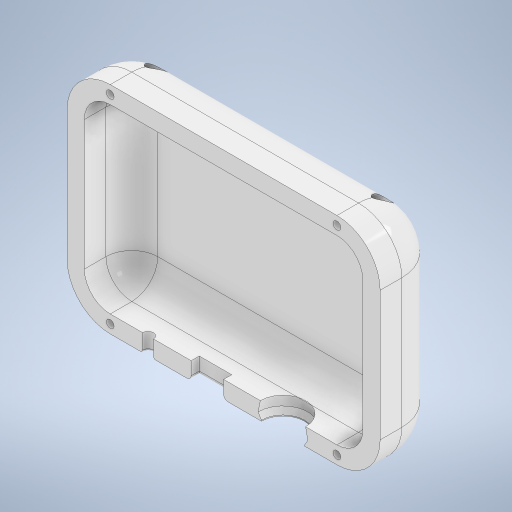
# Autodesk Inventor part: Case inferiore
Saved by Autodesk Inventor 2023 (Build 270158000, 158)
## iProperties
Created: 2022-12-30
Part Number: Case inferiore
Material: Plastica ABS
Document SubType Name: Modeling
Designer: Gabriele
Density: 1.06 g/cm^3
Appearance: Bianco
Author: Gabriele
Autodesk Inventor part; units mm, degrees
ref_plane "YZ Plane" through (0, 0, 0) normal (1, 0, 0) x (0, 1, 0)
ref_plane "XZ Plane" through (0, 0, 0) normal (0, 1, 0) x (-1, 0, 0)
ref_plane "XY Plane" through (0, 0, 0) normal (0, 0, 1) x (1, 0, 0)
sketch "Schizzo1" plane through (0, 0, 0) normal (0, 0, 1) x (1, 0, 0)
  line L0 (-52.5, -50) -> (52.5, -50)
  line L1 (72.5, -30) -> (72.5, 30)
  line L2 (52.5, 50) -> (-52.5, 50)
  line L3 (-72.5, 30) -> (-72.5, -30)
  line L4 (-72.5, -50) -> (72.5, 50) construction
  line L5 (72.5, -50) -> (-72.5, 50) construction
  arc A0 (-52.5, 50) -> (-72.5, 30) centre (-52.5, 30) ccw
  arc A1 (-72.5, -30) -> (-52.5, -50) centre (-52.5, -30) ccw
  arc A2 (52.5, -50) -> (72.5, -30) centre (52.5, -30) ccw
  arc A3 (72.5, 30) -> (52.5, 50) centre (52.5, 30) ccw
  point P0 (0, 0)
  dimension "d0" = 145
  dimension "d1" = 100
  dimension "d2" = 20
  constraints: 12 end point, 8 point on circle, 8 point on line, 8 tangent, 4 centre point, 3 equal radius, 2 midpoint, 2 parallel, 1 horizontal, 1 perpendicular
  measures "d0" distance of L4.end L5.end
  measures "d1" distance of L5.end L4.start
  measures "d2" radius of A0
extrude "Estrusione1" add sketch "Schizzo1" along normal blind 30
fillet "Raccordo1" radius 20 8 edges at (-66.6421, 44.1421, 0) (-72.5, 0, 0) (-66.6421, -44.1421, 0) (0, -50, 0) (66.6421, -44.1421, 0) (72.5, 0, 0) (66.6421, 44.1421, 0) (0, 50, 0)
shell "Svuotamento1" thickness 8 removed faces 1 at (17.5, 16.6667, 30)
sketch "Schizzo5" plane through (-52.5, -50, 30) normal (0, -1, 0) x (1, 0, 0)
  line L0 (52.5, 3.75) -> (37.5, 3.75)
  line L1 (37.5, 3.75) -> (37.5, -3.75)
  line L2 (37.5, -3.75) -> (52.5, -3.75)
  line L3 (52.5, -3.75) -> (52.5, 3.75)
  line L4 (105, 0) -> (0, 0) projected
  line L5 (52.5, 3.75) -> (37.5, -3.75) construction
  line L6 (37.5, 3.75) -> (52.5, -3.75) construction
  circle A0 centre (80, 0) radius 10
  circle A1 centre (17.5, 0) radius 2.55
  line L7 (0, 0) -> (105, 0) projected
  point P0 (52.5, -30)
  point P1 (52.5, 0)
  point P2 (52.5, 0)
  point P3 (70, 0)
  point P4 (90, 0)
  point P5 (52.5, 0)
  point P6 (37.5, 0)
  point P7 (14.95, 0)
  point P8 (20.05, 0)
  point P9 (45, 0)
  dimension "d16" = 5.1
  dimension "d17" = 15
  dimension "d19" = 20
  dimension "d28" = 3.75
  dimension "d29" = 7.5
  dimension "d78" = 25
  dimension "d79" = 27.5
  dimension "d80" = 17.5
  constraints: 12 end point, 4 point on line, 3 midpoint, 2 centre point, 2 parallel, 1 horizontal, 1 perpendicular
  measures "d16" diameter of A1
  measures "d17" distance of L0.start L0.end
  measures "d19" diameter of A0
  measures "d28" distance between parallel lines of L4 L2
  measures "d29" distance between parallel lines of L2 L0
  measures "d78" distance of L4.start A0.centre
  measures "d79" horizontal distance of L0.start A0.centre
  measures "d80" distance of L4.end A1.centre
extrude "Estrusione3" cut sketch "Schizzo5" against normal blind 9 contours L3 L2 L1 L4 | A0 L4 | A1 L4 picked at (77.0485, -1.5491) picked at (16.9445, -1.298)
sketch "Schizzo10" plane through (0, 0, 0) normal (0, 0, -1) x (-1, 0, 0)
  line L0 (52.5, 50) -> (-52.5, 50) projected
  line L1 (-72.5, 30) -> (-72.5, -30) projected
  line L2 (-52.5, -50) -> (-27.5, -50) projected
  line L3 (-27.5, -50) -> (52.5, -50) projected
  point P0 (0, 0)
  point P1 (52.5, 46)
  point P2 (-52.5, 46)
  point P3 (-52.5, -46)
  point P4 (52.5, -46)
  dimension "d69" = 4
  dimension "d70" = 4
  dimension "d71" = 20
  dimension "d72" = 105
  dimension "d74" = 105
  dimension "d75" = 20
  dimension "d76" = 4
  dimension "d77" = 4
  measures "d69" distance from line of L0 point (52.5, 46)
  measures "d70" distance from line of L0 point (-52.5, 46)
  measures "d71" distance from line of L1 point (-52.5, 46)
  measures "d72" distance of point (52.5, 46) point (-52.5, 46)
  measures "d74" distance of point (-52.5, -46) point (52.5, -46)
  measures "d75" distance from line of L1 point (-52.5, -46)
  measures "d76" distance from line of L2 point (-52.5, -46)
  measures "d77" distance from line of L3 point (52.5, -46)
hole "Foro5" at (-52.5, 46, 0) at (52.5, 46, 0) at (52.5, -46, 0) at (-52.5, -46, 0) direction (0, 0, 1) diameter 3.6 end through all counterbore diameter 6 counterbore depth 14 clearance for "Vite a testa esagonale con calotta ISO 24014 (Lamato/a)" size "M3" standard "ISO"
fillet "Raccordo2" radius 2 3 edges at (0, -50, 28.125) (-7.5, -50, 26.25) (-15, -50, 28.125)
fillet "Raccordo3" radius 1 1 edges at (-35, -50, 27.45)
sketch "Schizzo16" plane through (0, 0, 30) normal (0, 0, 1) x (1, 0, 0)
  line L0 (37.25, -50) -> (39, -47) projected
  line L1 (39, -47) -> (36.5, -34.5) projected
  line L2 (-52.5, -42) -> (52.5, -42) projected
  line L3 (-52.5, -50) -> (52.5, -50) projected
  line L4 (27.5, -50) -> (17.5, -50) projected
  line L5 (27.5, -50) -> (27.5, -42)
  point P0 (0, 0)
  point P1 (38, -42)
  constraints: 2 end point, 1 point on line, 1 vertical
revolve "Rivoluzione1" cut sketch "Schizzo16" angle 360 about axis through (27.5, -50, 30) along (0, 1, 0)
sketch "Schizzo17" plane through (0, 0, 0) normal (0, 0, -1) x (-1, 0, 0)
  line L0 (-52.5, 30) -> (52.5, 30) projected
  line L1 (-52.5, 30) -> (52.5, 30) projected
  line L2 (-52.5, -30) -> (-52.5, 30) projected
  line L3 (52.5, -30) -> (-52.5, -30) projected
  line L4 (52.5, 30) -> (52.5, -30) projected
  point P0 (0, 0)
extrude "Estrusione9" cut sketch "Schizzo17" against normal blind 2
